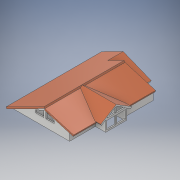
# Autodesk Inventor part: Dachgeschoss
Saved by Autodesk Inventor 2019 (Build 230136000, 136)
## iProperties
Created: 2019-04-30
Part Number: Dachgeschoss
Material: Generic
Document SubType Name: Modeling
Designer: niede
Density: 1 g/cm^3
Appearance: Default
Author: niede
Autodesk Inventor part; units mm, degrees
sketch "Skizze1" plane through (0, 0, 0) normal (0, 1, 0) x (-1, 0, 0)
  line L0 (0, 0) -> (11230, 0)
  line L1 (11230, 0) -> (11230, -6920)
  line L2 (11230, -6920) -> (10230, -6920)
  line L3 (10230, -6920) -> (10230, -17740)
  line L4 (10230, -17740) -> (11230, -17740)
  line L5 (11230, -17740) -> (11230, -17980)
  line L6 (11230, -17980) -> (2740, -17980)
  line L7 (2740, -17980) -> (2740, -14980)
  line L8 (2740, -14980) -> (-1250, -14980)
  line L9 (-1250, -14980) -> (-1250, -9110)
  line L10 (-1250, -9110) -> (-2000, -9110)
  line L11 (-2000, -9110) -> (-2000, -5010)
  line L12 (-2000, -5010) -> (0, -5010)
  line L13 (0, -5010) -> (0, 0)
  line L14 (1370, -5250) -> (-1760, -5250)
  line L15 (-1760, -5250) -> (-1760, -8870)
  line L16 (-1760, -8870) -> (1370, -8870)
  line L17 (1370, -8870) -> (1370, -5250)
  line L18 (9990, -17740) -> (7099.2495, -17740)
  line L19 (4780, -14980) -> (4780, -13169.8635)
  line L20 (4780, -13169.8635) -> (9990, -13169.8635)
  line L21 (9990, -13169.8635) -> (9990, -17740)
  line L22 (4780, -14980) -> (2980, -14980)
  line L23 (2980, -14980) -> (2980, -17740)
  line L24 (2980, -17740) -> (7099.2495, -17740)
  line L25 (2980, -14980) -> (2740, -14980)
  line L26 (9990, -13169.8635) -> (10230, -13169.8635)
  line L27 (10230, -17740) -> (9990, -17740)
  line L28 (9990, -17740) -> (9990, -17980)
  line L29 (2980, -17740) -> (2740, -17740)
  line L30 (2980, -17740) -> (2980, -17980)
  line L31 (9990, -17740) -> (2980, -17740)
  dimension "d0" = 11230
  dimension "d1" = 6920
  dimension "d2" = 1000
  dimension "d3" = 10820
  dimension "d4" = 1000
  dimension "d5" = 240
  dimension "d6" = 8490
  dimension "d7" = 3000
  dimension "d8" = 3990
  dimension "d9" = 5870
  dimension "d10" = 750
  dimension "d11" = 4100
  dimension "d12" = 2000
  dimension "d13" = 11230
  dimension "d14" = 6920
  dimension "d138" = 3370
  dimension "d139" = 240
  dimension "d140" = 240
  dimension "d141" = 240
  dimension "d142" = 240
  dimension "d143" = 240
  dimension "d144" = 240
  dimension "d145" = 4570.1365
  dimension "d146" = 2760
  dimension "d147" = 5210
  constraints: 64 end point, 14 perpendicular, 8 point on line, 5 parallel, 4 horizontal, 2 vertical, 1 collinear
  measures "d0" distance of L0.start L0.end
  measures "d1" distance of L0.end L1.end
  measures "d2" distance of L1.end L2.end
  measures "d3" distance of L2.end L3.end
  measures "d4" distance of L3.end L4.end
  measures "d5" distance of L4.end L5.end
  measures "d6" distance of L5.end L6.end
  measures "d7" distance of L6.end L7.end
  measures "d8" distance of L7.end L8.end
  measures "d9" distance of L8.end L9.end
  measures "d10" distance of L9.end L10.end
  measures "d11" distance of L10.end L11.end
  measures "d12" distance of L11.end L12.end
  measures "d13" distance from line of point (0, 0) L1
  measures "d14" distance from line of point (0, 0) L2
  measures "d138" distance between parallel lines of L17 L11
  measures "d139" distance between parallel lines of L11 L15
  measures "d140" distance between parallel lines of L12 L14
  measures "d141" distance between parallel lines of L10 L16
  measures "d142" distance between parallel lines of L7 L23
  measures "d143" distance between parallel lines of L6 L24
  measures "d144" distance between parallel lines of L3 L21
  measures "d145" distance between parallel lines of L18 L20
  measures "d146" distance between parallel lines of L24 L22
  measures "d147" distance of L19.end L20.end
extrude "Fundament" add sketch "Skizze1" along normal blind 300 contours L0 L1 L2 L3 L26 L20 L19 L22 L25 L8 L9 L10 L11 L12 L13 | L3 L27 L21 L26 | L4 L5 L6 L28 L27 | L28 L6 L30 L24 L18 | L25 L23 L29 L7 | L29 L30 L6 L7
sketch "Skizze3" plane through (0, 300, 0) normal (0, 1, 0) x (1, 0, 0)
  line L0 (-1370, 5250) -> (-1370, 8870) projected
  line L1 (-1370, 8870) -> (1760, 8870) projected
  line L2 (1760, 8870) -> (1760, 5250) projected
  line L3 (1760, 5250) -> (-1370, 5250) projected
  line L4 (-9990, 13169.8635) -> (-9990, 17740) projected
  line L5 (-9990, 17740) -> (-2980, 17740) projected
  line L6 (-2980, 14980) -> (-4780, 14980) projected
  line L7 (-4780, 14980) -> (-4780, 13169.8635) projected
  line L8 (-4780, 13169.8635) -> (-9990, 13169.8635) projected
  line L9 (-10230, 17740) -> (-10230, 6920) projected
  line L10 (-10230, 6920) -> (-11230, 6920) projected
  line L11 (-11230, 6920) -> (-11230, 0) projected
  line L12 (-11230, 0) -> (0, 0) projected
  line L13 (0, 0) -> (0, 5010) projected
  line L14 (0, 5010) -> (2000, 5010) projected
  line L15 (2000, 5010) -> (2000, 9110) projected
  line L16 (1250, 9110) -> (1250, 14980) projected
  line L17 (1250, 14980) -> (-2740, 14980) projected
  line L18 (-2740, 14980) -> (-2740, 17980) projected
  line L19 (-2740, 17980) -> (-11230, 17980) projected
  line L20 (-11230, 0) -> (-11230, 6920)
  line L21 (-10230, 6920) -> (-10230, 17740)
  line L22 (-11230, 17740) -> (-11230, 17980)
  line L23 (-2740, 17980) -> (-2740, 14980)
  line L24 (1250, 14980) -> (-2740, 14980) projected
  line L25 (1250, 14980) -> (1250, 9110)
  line L26 (2000, 9110) -> (2000, 5010)
  line L27 (0, 5010) -> (0, 0)
  line L28 (-11230, 0) -> (0, 0)
  line L29 (-11230, 17980) -> (-2740, 17980)
  line L30 (-10230, 17740) -> (-11230, 17740)
  line L31 (-11230, 6920) -> (-10230, 6920)
  line L32 (0, 5010) -> (2000, 5010)
  line L33 (2000, 9110) -> (1250, 9110)
  line L34 (1250, 14980) -> (-2740, 14980)
  line L35 (-9990, 13169.8635) -> (-9990, 17740)
  line L36 (-2980, 17740) -> (-9990, 17740)
  line L37 (-4780, 13169.8635) -> (-9990, 13169.8635)
  line L38 (-2980, 14980) -> (-4780, 14980) projected
  line L39 (-4780, 14980) -> (-4780, 13169.8635) projected
  line L40 (-4780, 14740) -> (-4780, 13169.8635)
  line L41 (-4780, 14980) -> (-2980, 14980)
  line L42 (-2980, 14980) -> (-2980, 17740)
  line L43 (-1370, 5250) -> (-1370, 8870)
  line L44 (1760, 8870) -> (-1370, 8870) projected
  line L45 (-1370, 8870) -> (1760, 8870)
  line L46 (1760, 8870) -> (1760, 5250)
  line L47 (-1370, 5250) -> (1760, 5250)
  line L48 (-240, 5010) -> (-240, 240)
  line L49 (-240, 240) -> (-10990, 240)
  line L50 (-10990, 240) -> (-10990, 6680)
  line L51 (-10990, 6680) -> (-9990, 6680)
  line L52 (-9990, 6680) -> (-9990, 12929.8635)
  line L53 (-9990, 12929.8635) -> (-4540, 12929.8635)
  line L54 (-4540, 12929.8635) -> (-4540, 14740)
  line L55 (-4540, 14740) -> (1010, 14740)
  line L56 (1010, 14740) -> (1010, 9110)
  line L57 (1010, 9110) -> (-1610, 9110)
  line L58 (-1610, 9110) -> (-1610, 5010)
  line L59 (-1610, 5010) -> (-240, 5010)
  line L60 (-4780, 14740) -> (-7280, 14740)
  line L61 (-7280, 14740) -> (-7280, 14980)
  line L62 (-7280, 14980) -> (-4780, 14980)
  dimension "d150" = 240
  dimension "d151" = 240
  dimension "d152" = 240
  dimension "d153" = 240
  dimension "d154" = 240
  dimension "d155" = 240
  dimension "d156" = 240
  dimension "d157" = 240
  dimension "d158" = 240
  dimension "d159" = 240
  dimension "d160" = 240
  dimension "d161" = 240
  dimension "d244" = 240
  dimension "d245" = 2500
  constraints: 78 end point, 17 perpendicular, 15 collinear, 5 parallel, 2 horizontal
  measures "d150" distance between parallel lines of L12 L49
  measures "d151" distance between parallel lines of L11 L50
  measures "d152" distance between parallel lines of L10 L51
  measures "d153" distance between parallel lines of L9 L52
  measures "d154" distance between parallel lines of L8 L53
  measures "d155" distance between parallel lines of L7 L54
  measures "d156" distance between parallel lines of L6 L55
  measures "d157" distance between parallel lines of L16 L56
  measures "d158" distance between parallel lines of L1 L57
  measures "d159" distance between parallel lines of L0 L58
  measures "d160" distance between parallel lines of L3 L59
  measures "d161" distance between parallel lines of L13 L48
  measures "d244" distance between parallel lines of L62 L60
  measures "d245" distance of L40.start L60.end
extrude "Wände" add sketch "Skizze3" along normal blind 3100 contours L60 L61 L62 L7 | L30 L22 L19 L18 L17 L16 L33 L15 L14 L13 L12 L11 L10 L9
sketch "Skizze4" plane through (1250, 0, -9110) normal (1, 0, 0) x (0, 0, -1)
  line L0 (5870, 0) -> (5870, 3400) projected
  line L1 (0, 3400) -> (5870, 3400) projected
  line L2 (0, 300) -> (0, 3400) projected
  line L3 (0, 1700) -> (5870, 1700)
  point P0 (-9110, 0)
  constraints: 2 end point, 1 midpoint, 1 parallel, 1 point on line
extrude "Wand_Ost" cut sketch "Skizze4" against normal blind 240
ref_plane "Dach_Süd_Ebene" through (1250, 1700, -12045) normal (-0.2817177, -0.9594973, 0) x (0, 0, 1)
sketch "Skizze5" plane through (1250, 1700, -12045) normal (-0.2817177, -0.9594973, 0) x (0, 0, 1)
  line L0 (12345, 6007.5034) -> (-3235, 6007.5034)
  line L1 (-3235, 6007.5034) -> (-3235, -192.4966)
  line L2 (12345, 178.2918) -> (12345, 6007.5034)
  line L3 (12045, 12453.4468) -> (12045, 1678.2918) projected
  line L4 (-2935, 709.1994) -> (-2935, 4307.3145) projected
  line L5 (12045, 1678.2918) -> (7035, 1678.2918) projected
  line L6 (7035, 1678.2918) -> (7035, -240.7029) projected
  line L7 (7035, 178.2918) -> (7035, 3229.1037)
  line L8 (6795, 2992.8031) -> (3175, 2992.8031) projected
  line L9 (-3235, -192.4966) -> (3175, -192.4966)
  line L10 (6795, 178.2918) -> (12345, 178.2918)
  line L11 (6795, 178.2918) -> (6795, 2992.8031)
  line L12 (3175, 2992.8031) -> (3175, -10.4236) projected
  line L13 (6795, 2992.8031) -> (3175, 2992.8031)
  line L14 (3175, 2992.8031) -> (3175, -192.4966)
  point P0 (12045, 720.4516)
  dimension "d166" = 300
  dimension "d167" = 300
  dimension "d181" = 90
  dimension "d183" = 3014.7003
  dimension "d184" = 1550.812
  dimension "d185" = 6200
  dimension "d186" = 1500
  constraints: 18 end point, 7 perpendicular, 2 point on line, 1 horizontal, 1 vertical
  measures "d166" distance between parallel lines of L3 L2
  measures "d167" distance between parallel lines of L4 L1
  measures "d181" angle of L8 L7
  measures "d183" distance between parallel lines of L8 L0
  measures "d184" distance from line of L7.end L5
  measures "d185" distance of L0.end L1.end
  measures "d186" distance between parallel lines of L5 L10
extrude "Dach_Süd" add sketch "Skizze5" along normal blind 300
sketch "Skizze6" plane through (-1370, 0, -5250) normal (1, 0, 0) x (0, 0, -1)
  line L0 (3620, 0) -> (3620, 3400) projected
  line L1 (0, 3400) -> (3620, 3400) projected
  line L2 (-240, 0) -> (3860, 0) projected
  line L3 (2467.2865, 3400) -> (3860, 3400)
  line L4 (3860, 3400) -> (3860, 0)
  line L5 (3860, 0) -> (2467.2865, 0)
  line L6 (2467.2865, 0) -> (2467.2865, 3400)
  point P0 (-5250, 0)
  dimension "d176" = 1152.7135
  constraints: 8 end point, 2 parallel, 1 horizontal, 1 perpendicular, 1 point on line
  measures "d176" distance between parallel lines of L0 L6
extrude "Tür" cut sketch "Skizze6" against normal blind 300
sketch "Skizze8" plane through (1010, 3400, -14980) normal (0, 0, -1) x (-1, 0, 0)
  line L0 (0, -1629.5337) -> (3750, -528.4974) projected
  line L1 (3750, -528.4974) -> (3750, 0) projected
  line L2 (0, 0) -> (3750, 0) projected
  line L3 (0, 0) -> (0, -1629.5337) projected
  point P0 (1010, -3400)
extrude "Dach_Süd_Rechts" cut sketch "Skizze8" against normal blind 240
sketch "Skizze9" plane through (-11230, 0, 0) normal (0, 0, 1) x (1, 0, 0)
  line L0 (6715.8164, 3392.42) -> (11230, 2067.0121) projected
  line L1 (0, 3400) -> (11230, 3400) projected
  line L2 (11230, 3400) -> (6654.8302, 3400)
  line L3 (6715.8164, 3392.42) -> (6654.8302, 3400)
  line L4 (6715.8164, 3392.42) -> (11230, 2067.0121)
  line L5 (11230, 2067.0121) -> (11230, 3400)
  constraints: 8 end point, 1 perpendicular, 1 point on line
extrude "Dach_Süd_Verbesserung_1" cut sketch "Skizze9" against normal blind 5010
sketch "Skizze10" plane through (-4540, 3400, -14740) normal (0, 0, 1) x (1, 0, 0)
  line L0 (1800, -528.4974) -> (1800, 0) projected
  line L1 (0, 0) -> (1800, 0) projected
  line L2 (0, -95.5077) -> (0, 0) projected
  line L3 (0, -95.5077) -> (25.8164, -7.58) projected
  line L4 (25.8164, -7.58) -> (1800, -528.4974) projected
  point P0 (4540, -3400)
extrude "Dach_Süd_Verbesserung_2" cut sketch "Skizze10" against normal blind 5000
ref_plane "Dach_Nord_Ebene" through (-4514.1836, 3392.42, 300) normal (-0.4508793, 0.8925849, 0) x (0, 0, -1)
sketch "Skizze11" plane through (-4514.1836, 3392.42, 300) normal (-0.4508793, 0.8925849, 0) x (0, 0, -1)
  line L0 (0, -4251.8978) -> (0, 0) projected
  line L1 (0, 0) -> (15580, 0)
  line L2 (18580, 3600) -> (18580, 8291.0187)
  line L3 (18580, 8291.0187) -> (0, 8291.0187)
  line L4 (0, 8291.0187) -> (0, 0)
  line L5 (7220, 5991.0187) -> (300, 5991.0187) projected
  line L6 (18280, 19.6257) -> (18280, 5991.0187) projected
  line L7 (15580, 205.2223) -> (15580, -1025.3164) projected
  line L8 (15580, 0) -> (15580, 3600)
  line L9 (15580, 3600) -> (18580, 3600)
  point P0 (300, -2499.72)
  dimension "d193" = 2300
  dimension "d194" = 300
  dimension "d230" = 3600
  constraints: 12 end point, 2 parallel, 2 perpendicular, 1 collinear, 1 horizontal, 1 point on line
  measures "d193" distance between parallel lines of L3 L5
  measures "d194" distance between parallel lines of L6 L2
  measures "d230" distance of L1.end L8.end
extrude "Dach_Nord" add sketch "Skizze11" along normal blind 300
sketch "Skizze12" plane through (-11230, 3400, 0) normal (0, 0, 1) x (1, 0, 0)
  line L0 (0, -3063.8975) -> (6065.4557, 0) projected
  line L1 (0, 0) -> (6065.4557, 0) projected
  line L2 (0, -3063.8975) -> (0, 0) projected
  point P0 (11230, -3400)
extrude "Dach_Nord_Verbesserung_1" cut sketch "Skizze12" against normal blind 20000
sketch "Skizze13" plane through (2000, 0, -5010) normal (1, 0, 0) x (0, 0, -1)
  line L0 (4100, 0) -> (4100, 3400) projected
  line L1 (0, 0) -> (0, 3400) projected
  line L2 (-950, 1824.8148) -> (2050, 3660.1955)
  line L3 (-5310, 3660.1955) -> (10270, 3660.1955) projected
  line L4 (5050.0001, 1824.8149) -> (2050, 3660.1955)
  line L5 (-950, 1824.8148) -> (-949.9999, 1824.8147)
  line L6 (-4770, 1824.8147) -> (0, 1824.8147) projected
  line L7 (-949.9999, 1824.8147) -> (2050, 3660.1954)
  line L8 (2050, 3660.1954) -> (5050, 1824.8148)
  line L9 (10270, 1645.7703) -> (4100, 1645.7703) projected
  line L10 (5050.0001, 1824.8149) -> (5050, 1824.8148)
  line L11 (-949.9999, 1824.8147) -> (-793.4378, 1568.9079)
  line L12 (-793.4378, 1568.9079) -> (2050, 3308.5048)
  line L13 (2050, 3308.5048) -> (4893.4378, 1568.9079)
  line L14 (4893.4378, 1568.9079) -> (5050, 1824.8148)
  point P0 (-5010, 0)
  point P1 (13270, 3660.1955)
  dimension "d199" = 2050
  dimension "d200" = 3000
  dimension "d201" = 3000
  dimension "d202" = 2050
  dimension "d203" = 300
  dimension "d204" = 180
  dimension "d205" = 76.8624
  constraints: 20 end point, 4 perpendicular, 3 parallel, 2 equal length, 2 point on line
  measures "d199" distance from line of L1 L2.end
  measures "d200" horizontal distance of L2.start L7.end
  measures "d201" horizontal distance of L8.end L7.end
  measures "d202" distance from line of L0 L7.end
  measures "d203" distance of L5.end L11.end
  measures "d204" angle of L8 L13
  measures "d205" distance from line of L13.end L9
extrude "Dach_Süd_Spitze" add sketch "Skizze13" against normal blind 6650 contours L13 L12 L1 L2 L4 L0 | L0 L4 L14 L9 L13 | L9 L14 L13 | L12 L6 L2 L1 | L12 L11 L6
sketch "Skizze15" plane through (2000, 0, -5010) normal (1, 0, 0) x (0, 0, -1)
  line L0 (4100, 2406.0186) -> (4100, 3400) projected
  line L1 (2475.2993, 3400) -> (4100, 3400) projected
  line L2 (2050, 3660.1954) -> (1624.7007, 3400) projected
  line L3 (0, 3400) -> (1624.7007, 3400) projected
  line L4 (0, 2406.0185) -> (1624.7007, 3400)
  line L5 (1624.7007, 3400) -> (0, 3400) projected
  line L6 (0, 3400) -> (0, 2406.0185)
  line L7 (1624.7007, 3400) -> (240, 2552.849) projected
  line L8 (1624.7007, 3400) -> (0, 3400)
  line L9 (3860, 2552.8491) -> (2475.2993, 3400) projected
  line L10 (2475.2993, 3400) -> (4100, 3400)
  line L11 (4100, 2406.0186) -> (4100, 3400)
  line L12 (4100, 2406.0186) -> (3860, 2552.8491) projected
  line L13 (2475.2993, 3400) -> (4100, 2406.0186)
  point P0 (-5010, 0)
  constraints: 12 end point, 4 collinear, 1 perpendicular, 1 vertical
extrude "Dach_Süd_Spitze_Verbesserung_1" cut sketch "Skizze15" against normal blind 3610
sketch "Skizze22" plane through (-1154.6161, 2406.0185, -5010) normal (0, 0, -1) x (-1, 0, 0)
  line L0 (455.3839, 133.7051) -> (0, 0) projected
  line L1 (0, 0) -> (455.3839, 0) projected
  line L2 (455.3839, 0) -> (455.3839, 133.7051) projected
  point P0 (-1154.6161, -2406.0185)
extrude "Dach_Süd_Spitze_Verbesserung_2" add sketch "Skizze22" along normal blind 250
sketch "Skizze23" plane through (-1670, 2406.0186, -9110) normal (0, 0, 1) x (1, 0, 0)
  line L0 (0, 151.3216) -> (515.3835, 0) projected
  line L1 (0, 151.3216) -> (0, 0) projected
  line L2 (515.3835, 0) -> (0, 0) projected
  point P0 (1670, -2406.0186)
extrude "Dach_Süd_Spitze_Verbesserung_3" add sketch "Skizze23" along normal blind 250
sketch "Skizze16" plane through (2000, 0, -5010) normal (1, 0, 0) x (0, 0, -1)
  line L0 (5050, 1824.8148) -> (2050, 3660.1954) projected
  line L1 (2050, 3660.1954) -> (-949.9999, 1824.8147) projected
  line L2 (0, 0) -> (0, 2054.328) projected
  line L3 (0, 0) -> (4100, 0) projected
  line L4 (4100, 0) -> (4100, 2054.328) projected
  line L5 (1930, 1900) -> (240, 1900)
  line L6 (240, 1900) -> (240, 300)
  line L7 (240, 300) -> (1930, 300)
  line L8 (1930, 300) -> (1930, 1900)
  line L9 (2170, 1900) -> (3860, 1900)
  line L10 (3860, 1900) -> (3860, 300)
  line L11 (3860, 300) -> (2170, 300)
  line L12 (2170, 300) -> (2170, 1900)
  line L13 (3771.5422, 2255.2764) -> (328.4578, 2255.2764) projected
  line L14 (240, 2255.2764) -> (1956.1093, 3321.4012)
  line L15 (1956.1093, 3321.4012) -> (1956.1093, 2271.4967)
  line L16 (2707.2865, 2543.1256) -> (798.9583, 2543.1256) projected
  line L17 (1956.1093, 2271.4967) -> (266.1093, 2271.4967)
  line L18 (2170, 2271.4967) -> (2170, 3305.4277)
  line L19 (2170, 3305.4277) -> (3860, 2271.4967)
  line L20 (3860, 2271.4967) -> (2170, 2271.4967)
  point P0 (-5010, 0)
  dimension "d216" = 300
  dimension "d217" = 1600
  dimension "d218" = 240
  dimension "d219" = 240
  dimension "d220" = 240
  dimension "d221" = 1690
  dimension "d222" = 1690
  dimension "d223" = 240
  dimension "d224" = 240
  dimension "d225" = 1690
  dimension "d226" = 240
  dimension "d227" = 240
  constraints: 28 end point, 6 point on line, 5 parallel, 5 perpendicular, 2 horizontal, 1 vertical
  measures "d216" distance between parallel lines of L3 L7
  measures "d217" distance of L5.end L6.end
  measures "d218" distance between parallel lines of L4 L10
  measures "d219" distance between parallel lines of L2 L6
  measures "d220" distance between parallel lines of L12 L8
  measures "d221" distance of L10.end L11.end
  measures "d222" distance of L15.end L17.end
  measures "d223" distance from line of L2 L14.start
  measures "d224" distance from line of L4 L19.end
  measures "d225" distance of L19.end L18.start
  measures "d226" distance from line of L1 L14.end
  measures "d227" distance between parallel lines of L0 L19
extrude "Dach_Süd_Fenster" cut sketch "Skizze16" against normal blind 240
ref_plane "Dach_West_Ebene" through (-2740, 0, -14980) normal (0.3695023, 0.9292298, 0) x (0, 0, -1)
sketch "Skizze17" plane through (-2740, 0, -14980) normal (0.3695023, 0.9292298, 0) x (0, 0, -1)
  line L0 (3300, 5512.9021) -> (3300, 8622.1823) projected
  line L1 (3300, 5512.9021) -> (3300, -338.9733)
  line L2 (3300, -338.9733) -> (0, -338.9733)
  line L3 (0, 945.4968) -> (0, -3195.0031) projected
  line L4 (0, -338.9733) -> (0, 5512.9021)
  line L5 (0, 5512.9021) -> (3300, 5512.9021)
  line L6 (3000, 1061.0267) -> (300, 1061.0267) projected
  point P0 (-14980, -2546.0897)
  dimension "d231" = 1400
  constraints: 8 end point, 2 perpendicular, 2 vertical, 1 point on line
  measures "d231" distance between parallel lines of L6 L2
extrude "Dach_West" add sketch "Skizze17" against normal blind 300
sketch "Skizze19" plane through (-2980, 2629.3052, -15280) normal (0, 0, -1) x (-1, 0, 0)
  line L0 (1618.6989, 475.2656) -> (0, 0) projected
  line L1 (1534.1836, 763.1148) -> (0, 312.6637) projected
  line L2 (-1370, -89.5815) -> (1534.1836, 763.1148) projected
  line L3 (1618.6989, 475.2656) -> (1558.8219, 679.1996) projected
  line L4 (1534.1836, 763.1148) -> (1618.6989, 475.2656)
  line L5 (1618.6989, 475.2656) -> (-303.859, -89.2159)
  line L6 (-240, -70.4663) -> (-4230, -1241.9689) projected
  line L7 (-388.3743, 198.6333) -> (1534.1836, 763.1148)
  line L8 (-388.3743, 198.6333) -> (-303.859, -89.2159)
  line L9 (1248.3783, 679.1996) -> (-1358.4134, -86.1796) projected
  line L10 (1560, -2329.3052) -> (1560, 458.0311) projected
  line L11 (-303.859, -89.2159) -> (1560, 458.0311)
  point P0 (-2980, -2629.3052)
  dimension "d237" = 2003.7136
  constraints: 10 end point, 2 collinear, 2 perpendicular, 1 point on line
  measures "d237" distance between parallel lines of L3 L8
extrude "Dach_West_Verbesserung_1" cut sketch "Skizze19" along normal blind 3000
sketch "Skizze20" plane through (-4514.1836, 3392.42, -15280) normal (0, 0, -1) x (-0.8925849, -0.4508793, 0)
  line L0 (3334.4428, 0) -> (3600, 300) projected
  line L1 (0, 300) -> (3600, 300) projected
  line L2 (0, 0) -> (0, 300) projected
  line L3 (0, 0) -> (3334.4428, 0) projected
  point P0 (-2499.72, -5063.3751)
extrude "Dach_West_Verbesserung_2" cut sketch "Skizze20" along normal blind 3000
sketch "Skizze21" plane through (-2980, 95.4345, -14980) normal (0, 0, -1) x (-1, 0, 0)
  line L0 (0, 0) -> (4300, 1709.8674) projected
  line L1 (1800, -95.4345) -> (1800, 204.5655) projected
  line L2 (4300, 1899.8641) -> (1560, 3283.9447) projected
  line L3 (1560, 3283.9447) -> (1560, 3209.0578) projected
  line L4 (1560, 3209.0578) -> (1618.6989, 3009.1364) projected
  line L5 (1618.6989, 3009.1364) -> (0, 2533.8707) projected
  line L6 (0, 0) -> (0, 2533.8707) projected
  line L7 (-240, -95.4345) -> (-240, 2463.4044) projected
  line L8 (-240, 2463.4044) -> (-240, -95.4345)
  line L9 (-240, -95.4345) -> (4510.4568, 1793.5542)
  line L10 (1534.1836, 3296.9856) -> (4510.4568, 1793.5542) projected
  line L11 (4510.4568, 1793.5542) -> (1534.1836, 3296.9856)
  line L12 (1534.1836, 3296.9856) -> (1618.6989, 3009.1364)
  line L13 (-240, 2463.4044) -> (-4230, 1291.9018) projected
  line L14 (1618.6989, 3009.1364) -> (-240, 2463.4044)
  point P0 (1800, 715.7585)
  point P1 (1800, 3162.7114)
  point P2 (-2980, -95.4345)
  constraints: 10 end point, 2 collinear, 1 vertical
extrude "Dach_West_Verbesserung_3" cut sketch "Skizze21" along normal blind 3000
sketch "Skizze24" plane through (0, 0, 0) normal (0, 0, 1) x (1, 0, 0)
  line L0 (-4514.1836, 3392.42) -> (-11230, 0) projected
  line L1 (0, 0) -> (0, 1754.3484) projected
  line L2 (0, 1754.3484) -> (-4598.6989, 3104.5708) projected
  line L3 (-5001.2237, 1498.2605) -> (-5001.2237, 2698.2605)
  line L4 (-5001.2237, 2698.2605) -> (-6601.2237, 2012.7367)
  line L5 (-6601.2237, 2012.7367) -> (-6601.2237, 1498.2605)
  line L6 (-6601.2237, 1498.2605) -> (-5001.2237, 1498.2605)
  line L7 (-4601.2237, 2698.2605) -> (-4601.2237, 1498.2605)
  line L8 (-4601.2237, 1498.2605) -> (-3001.2237, 1498.2605)
  line L9 (-3001.2237, 1498.2605) -> (-3001.2237, 2012.7367)
  line L10 (-3001.2237, 2012.7367) -> (-4601.2237, 2698.2605)
  dimension "d250" = 400
  dimension "d251" = 1600
  dimension "d252" = 1200
  dimension "d253" = 400
  dimension "d254" = 6.83
  dimension "d255" = 3001.2238
  constraints: 16 end point, 3 equal length, 3 perpendicular, 2 point on line, 1 parallel, 1 vertical
  measures "d250" distance between parallel lines of L7 L3
  measures "d251" distance of L5.end L3.start
  measures "d252" distance of L3.start L3.end
  measures "d253" distance from line of L0 L3.end
  measures "d254" angle of L2 L10
  measures "d255" distance between parallel lines of L1 L9
extrude "Fenster_West" cut sketch "Skizze24" against normal blind 240
sketch "Skizze25" plane through (1250, 0, -14980) normal (0, 0, -1) x (-1, 0, 0)
  line L0 (5848.6989, 3104.5708) -> (0, 1387.3363) projected
  line L1 (8530, 1805.3019) -> (8530, 1995.2986) projected
  line L2 (2961.6445, 944.24) -> (3961.6445, 944.24)
  line L3 (3961.6445, 944.24) -> (3961.6445, 1144.24)
  line L4 (3961.6445, 1144.24) -> (4961.6445, 1144.24)
  line L5 (4961.6445, 1144.24) -> (4961.6445, 2144.24)
  line L6 (4961.6445, 2144.24) -> (4361.6445, 2355.2936)
  line L7 (2961.6445, 944.24) -> (2961.6445, 1944.24)
  line L8 (1490, 1568.9079) -> (5900, 1568.9079) projected
  line L9 (2961.6445, 1944.24) -> (4361.6445, 2355.2936)
  line L10 (5848.6989, 3104.5708) -> (-100.1846, 1357.9211) projected
  point P0 (1250, 0)
  dimension "d258" = 300
  dimension "d259" = 1000
  dimension "d260" = 1000
  dimension "d261" = 1400
  dimension "d262" = 200
  dimension "d263" = 3568.3555
  constraints: 14 end point, 4 perpendicular, 3 parallel, 1 horizontal
  measures "d258" distance between parallel lines of L0 L9
  measures "d259" distance of L2.start L7.end
  measures "d260" distance of L2.start L2.end
  measures "d261" horizontal distance of L7.end L6.end
  measures "d262" distance of L2.end L3.end
  measures "d263" distance between parallel lines of L1 L5
extrude "Fenster_ost" cut sketch "Skizze25" against normal blind 240
